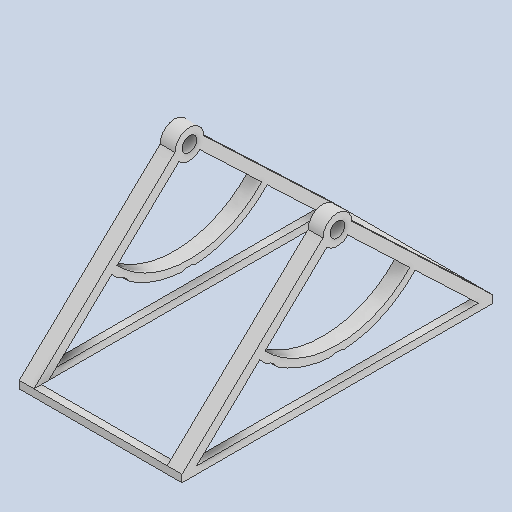
# Autodesk Inventor part: Cage2
Saved by Autodesk Inventor 2025 (Build 290162000, 162)
## iProperties
Created: 2025-08-06
Part Number: Cage2
Material: Generic
Document SubType Name: Modeling
Designer: Pravoslav
Density: 1 g/cm^3
Appearance: Default
Author: Pravoslav
Autodesk Inventor part; units mm, degrees
ref_plane "YZ Plane" through (0, 0, 0) normal (1, 0, 0) x (0, 1, 0)
ref_plane "XZ Plane" through (0, 0, 0) normal (0, 1, 0) x (-1, 0, 0)
ref_plane "XY Plane" through (0, 0, 0) normal (0, 0, 1) x (1, 0, 0)
sketch "Sketch1" plane through (0, 0, 0) normal (0, 1, 0) x (-1, 0, 0)
  line L0 (20, 40) -> (-20, 40)
  line L1 (-20, 40) -> (-20, -40)
  line L2 (-20, -40) -> (20, -40)
  line L3 (20, -40) -> (20, 40)
  line L4 (20, 40) -> (-20, -40) construction
  line L5 (-20, 40) -> (20, -40) construction
  line L6 (22, 42) -> (-22, 42)
  line L7 (-22, 42) -> (-22, -42)
  line L8 (-22, -42) -> (22, -42)
  line L9 (22, -42) -> (22, 42)
  line L10 (22, 42) -> (-22, -42) construction
  line L11 (-22, 42) -> (22, -42) construction
  point P0 (0, 0)
  dimension "d0" = 40
  dimension "d1" = 80
  dimension "d2" = 44
  dimension "d3" = 84
  constraints: 24 end point, 4 midpoint, 4 parallel, 2 horizontal, 2 perpendicular
  measures "d0" distance of L2.end L1.end
  measures "d1" distance between parallel lines of L2 L0
  measures "d2" distance of L8.end L7.end
  measures "d3" distance of L7.end L6.end
extrude "Extrusion1" add sketch "Sketch1" along normal blind 2
sketch "Sketch2" plane through (-22, 0, -42) normal (-1, 0, 0) x (0, 0, 1)
  line L0 (2, 2) -> (82, 2) projected
  line L1 (42, 2) -> (42, 42)
  line L2 (0, 0) -> (0, 2) projected
  line L3 (42, 42) -> (0, 2)
  line L4 (0, 2) -> (2.087, 2)
  line L5 (84, 2) -> (0, 2) projected
  line L6 (42, 42) -> (84, 2)
  line L7 (3.9048, 2) -> (42, 38.2812)
  line L8 (42, 38.2812) -> (80.0952, 2)
  circle A0 centre (42, 38.2812) radius 2
  arc A1 (45.9048, 38.2812) -> (38.0952, 38.2812) centre (42, 38.2812) ccw
  circle A2 centre (42, 38.2812) radius 29
  circle A3 centre (42, 38.2812) radius 27
  arc A4 (44, 9.3502) -> (40.1623, 9.3395) centre (42.0932, 5.0544) ccw
  arc A5 (61.2326, 16.5762) -> (58.2295, 14.2478) centre (62.3651, 12.0146) ccw
  circle A6 centre (42, 38.2812) radius 3.9048
  point P0 (42, 0)
  point P1 (22.4483, 19.6605)
  point P2 (40.5517, 36.9019)
  point P3 (43.4483, 36.9019)
  point P4 (61.5517, 19.6605)
  point P5 (2, 2)
  point P6 (3.9048, 2)
  point P7 (21, 18.2812)
  point P8 (63, 18.2812)
  point P9 (80.0952, 2)
  point P10 (39.1724, 35.5882)
  point P11 (44.8276, 35.5882)
  dimension "d6" = 40
  dimension "d7" = 4
  dimension "d8" = 58
  dimension "d9" = 54
  dimension "d10" = 4.7
  dimension "d12" = 3.8
  dimension "d13" = 4.7
  constraints: 12 end point, 10 point on circle, 7 centre point, 5 point on line, 4 coincident, 2 parallel, 1 concentric, 1 midpoint, 1 perpendicular, 1 vertical
  measures "d6" distance of L1.start L1.end
  measures "d7" diameter of A0
  measures "d8" diameter of A2
  measures "d9" diameter of A3
  measures "d10" radius of A4
  measures "d12" distance of A5.end A5.start
  measures "d13" radius of A5
extrude "Extrusion2" add sketch "Sketch2" against normal blind 4 contours L4 L3 A2 L7 L0 | L3 A3 L7 A2 | L7 A3 L1 A4 A2 | L3 A6 L7 A3 | L8 A2 L6 L5 L0 | A1 L6 L3 | L3 L1 A0 L7 A6 | A2 L8 A3 L6 | A2 A5 A4 L1 A3 L8 | L7 A0 L1 A6 | L6 A6 L8 A0 L1 | L6 A3 L8 A6 | L1 A0 L8 A6
mirror "Mirror1" about plane through (0, 0, 0) normal (1, 0, 0) of "Extrusion2"
body "Solid1"
